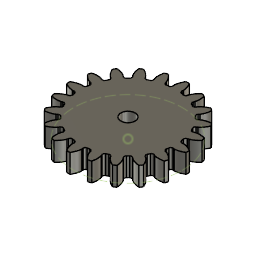
gear (Autodesk Fusion 360 design; units mm, degrees)
description: Spur Gear; Module: 2.000000; Num Teeth: 20; Pressure Angle: 20.000000; Backlash: 0.20 mm
Autodesk Fusion 360 part; units mm, degrees
(part 1 of 3)
sketch "Sketch1" plane through (0, 0, 0) normal (0, 0, 1) x (1, 0, 0) in component "Spur Gear (20 teeth)"
  circle A0 centre (0, 0) radius 17.5492
extrude "Extrude1" add sketch "Sketch1" along normal blind 7 in component "Spur Gear (20 teeth)"
sketch "Sketch2" plane through (0, 0, 0) normal (0, 0, 1) x (1, 0, 0) in component "Spur Gear (20 teeth)"
  spline S0 degree 5 poles (18.7162, -1.7068) (18.7256, -1.7077) (18.7444, -1.7091) (18.7726, -1.7106) (18.8102, -1.7111) (18.8573, -1.7097) (18.9045, -1.707) (18.9518, -1.7034) (18.999, -1.6994) (19.0463, -1.695) (19.0936, -1.6902) (19.1409, -1.6851) (19.1883, -1.6793) (19.2356, -1.6729) (19.2829, -1.6658) (19.3303, -1.658) (19.3776, -1.6497) (19.425, -1.641) (19.4723, -1.6318) (19.5197, -1.6223) (19.567, -1.6124) (19.6143, -1.6021) (19.6616, -1.5914) (19.7089, -1.5802) (19.7562, -1.5687) (19.8035, -1.5567) (19.8507, -1.5444) (19.898, -1.5316) (19.9452, -1.5186) (19.9924, -1.5051) (20.0396, -1.4914) (20.0867, -1.4773) (20.1339, -1.4628) (20.181, -1.448) (20.2281, -1.4329) (20.2752, -1.4174) (20.3222, -1.4016) (20.3692, -1.3854) (20.4162, -1.369) (20.4631, -1.3523) (20.5101, -1.3352) (20.557, -1.3178) (20.6038, -1.3001) (20.6506, -1.2822) (20.6974, -1.2639) (20.7442, -1.2453) (20.7909, -1.2264) (20.8376, -1.2073) (20.8843, -1.1878) (20.9309, -1.1681) (20.9774, -1.1481) (21.024, -1.1278) (21.0705, -1.1072) (21.1169, -1.0863) (21.1633, -1.0652) (21.2097, -1.0438) (21.256, -1.0221) (21.3023, -1.0002) (21.3485, -0.978) (21.3947, -0.9555) (21.4409, -0.9328) (21.487, -0.9098) (21.533, -0.8865) (21.579, -0.863) (21.625, -0.8392) (21.6709, -0.8151) (21.7167, -0.7909) (21.7625, -0.7663) (21.8083, -0.7415) (21.8539, -0.7165) (21.8996, -0.6912) (21.9361, -0.6707) (21.9634, -0.6553) (21.9816, -0.645) (21.9907, -0.6398) knots 0 0 0 0 0 0 0.01428571 0.02857143 0.04285714 0.05714286 0.07142857 0.08571429 0.1 0.11428571 0.12857143 0.14285714 0.15714286 0.17142857 0.18571429 0.2 0.21428571 0.22857143 0.24285714 0.25714286 0.27142857 0.28571429 0.3 0.31428571 0.32857143 0.34285714 0.35714286 0.37142857 0.38571429 0.4 0.41428571 0.42857143 0.44285714 0.45714286 0.47142857 0.48571429 0.5 0.51428571 0.52857143 0.54285714 0.55714286 0.57142857 0.58571429 0.6 0.61428571 0.62857143 0.64285714 0.65714286 0.67142857 0.68571429 0.7 0.71428571 0.72857143 0.74285714 0.75714286 0.77142857 0.78571429 0.8 0.81428571 0.82857143 0.84285714 0.85714286 0.87142857 0.88571429 0.9 0.91428571 0.92857143 0.94285714 0.95714286 0.97142857 0.98571429 1 1 1 1 1 1
  spline S1 degree 5 poles (18.7162, 1.7068) (18.7256, 1.7077) (18.7444, 1.7091) (18.7726, 1.7106) (18.8102, 1.7111) (18.8573, 1.7097) (18.9045, 1.707) (18.9518, 1.7034) (18.999, 1.6994) (19.0463, 1.695) (19.0936, 1.6902) (19.1409, 1.6851) (19.1883, 1.6793) (19.2356, 1.6729) (19.2829, 1.6658) (19.3303, 1.658) (19.3776, 1.6497) (19.425, 1.641) (19.4723, 1.6318) (19.5197, 1.6223) (19.567, 1.6124) (19.6143, 1.6021) (19.6616, 1.5914) (19.7089, 1.5802) (19.7562, 1.5687) (19.8035, 1.5567) (19.8507, 1.5444) (19.898, 1.5316) (19.9452, 1.5186) (19.9924, 1.5051) (20.0396, 1.4914) (20.0867, 1.4773) (20.1339, 1.4628) (20.181, 1.448) (20.2281, 1.4329) (20.2752, 1.4174) (20.3222, 1.4016) (20.3692, 1.3854) (20.4162, 1.369) (20.4631, 1.3523) (20.5101, 1.3352) (20.557, 1.3178) (20.6038, 1.3001) (20.6506, 1.2822) (20.6974, 1.2639) (20.7442, 1.2453) (20.7909, 1.2264) (20.8376, 1.2073) (20.8843, 1.1878) (20.9309, 1.1681) (20.9774, 1.1481) (21.024, 1.1278) (21.0705, 1.1072) (21.1169, 1.0863) (21.1633, 1.0652) (21.2097, 1.0438) (21.256, 1.0221) (21.3023, 1.0002) (21.3485, 0.978) (21.3947, 0.9555) (21.4409, 0.9328) (21.487, 0.9098) (21.533, 0.8865) (21.579, 0.863) (21.625, 0.8392) (21.6709, 0.8151) (21.7167, 0.7909) (21.7625, 0.7663) (21.8083, 0.7415) (21.8539, 0.7165) (21.8996, 0.6912) (21.9361, 0.6707) (21.9634, 0.6553) (21.9816, 0.645) (21.9907, 0.6398) knots 0 0 0 0 0 0 0.01428571 0.02857143 0.04285714 0.05714286 0.07142857 0.08571429 0.1 0.11428571 0.12857143 0.14285714 0.15714286 0.17142857 0.18571429 0.2 0.21428571 0.22857143 0.24285714 0.25714286 0.27142857 0.28571429 0.3 0.31428571 0.32857143 0.34285714 0.35714286 0.37142857 0.38571429 0.4 0.41428571 0.42857143 0.44285714 0.45714286 0.47142857 0.48571429 0.5 0.51428571 0.52857143 0.54285714 0.55714286 0.57142857 0.58571429 0.6 0.61428571 0.62857143 0.64285714 0.65714286 0.67142857 0.68571429 0.7 0.71428571 0.72857143 0.74285714 0.75714286 0.77142857 0.78571429 0.8 0.81428571 0.82857143 0.84285714 0.85714286 0.87142857 0.88571429 0.9 0.91428571 0.92857143 0.94285714 0.95714286 0.97142857 0.98571429 1 1 1 1 1 1
  arc A0 (21.9907, -0.6398) -> (21.9907, 0.6398) centre (0, 0) ccw
  line L0 (17.4667, -1.5938) -> (18.7162, -1.7068)
  line L1 (17.4667, 1.5938) -> (18.7162, 1.7068)
  line L2 (17.4667, -1.5938) -> (17.4667, 1.5938)
  point P0 (18.9464, -1.7037)
  point P1 (19.1784, -1.6804)
  point P2 (19.4114, -1.6434)
  point P3 (19.6452, -1.595)
  point P4 (19.8796, -1.5365)
  point P5 (20.1144, -1.4687)
  point P6 (20.3494, -1.3922)
  point P7 (20.5845, -1.3074)
  point P8 (20.8195, -1.2147)
  point P9 (21.0545, -1.1142)
  point P10 (21.2892, -1.0064)
  point P11 (21.5235, -0.8912)
  point P12 (21.7574, -0.769)
  point P13 (18.9464, 1.7037)
  point P14 (19.1784, 1.6804)
  point P15 (19.4114, 1.6434)
  point P16 (19.6452, 1.595)
  point P17 (19.8796, 1.5365)
  point P18 (20.1144, 1.4687)
  point P19 (20.3494, 1.3922)
  point P20 (20.5845, 1.3074)
  point P21 (20.8195, 1.2147)
  point P22 (21.0545, 1.1142)
  point P23 (21.2892, 1.0064)
  point P24 (21.5235, 0.8912)
  point P25 (21.7574, 0.769)
extrude "Extrude2" add sketch "Sketch2" along normal blind 7 in component "Spur Gear (20 teeth)"
fillet "Fillet1" radius 0.75 2 edges at (17.4766, -1.5947, 3.5) (17.4766, 1.5947, 3.5) in component "Spur Gear (20 teeth)"
pattern_circular "C-Pattern1" count 20 over 360 about axis through (0, 0, 0) along (0, 0, 1) of "Extrude2", "Fillet1" in component "Spur Gear (20 teeth)"
sketch "Sketch3" plane through (0, 0, 0) normal (0, 0, 1) x (1, 0, 0) in component "Spur Gear (20 teeth)"
  circle A0 centre (0, 0) radius 20 construction
sketch "Sketch1 (2)" plane through (0, 0, 7) normal (0, 0, 1) x (-1, 0, 0)
  arc A0 (-17.2587, 3.1798) -> (-17.3966, 2.3091) centre (0, 0) ccw
  arc A1 (-18.2077, 1.6608) -> (-17.3966, 2.3091) centre (-18.1401, 2.4078) ccw
  line L0 (-18.2077, 1.6608) -> (-18.7162, 1.7068)
  spline S0 degree 5 poles (-18.7162, 1.7068) (-18.7256, 1.7077) (-18.7444, 1.7091) (-18.7726, 1.7106) (-18.8102, 1.7111) (-18.8573, 1.7097) (-18.9045, 1.707) (-18.9518, 1.7034) (-18.999, 1.6994) (-19.0463, 1.695) (-19.0936, 1.6902) (-19.1409, 1.6851) (-19.1883, 1.6793) (-19.2356, 1.6729) (-19.2829, 1.6658) (-19.3303, 1.658) (-19.3776, 1.6497) (-19.425, 1.641) (-19.4723, 1.6318) (-19.5197, 1.6223) (-19.567, 1.6124) (-19.6143, 1.6021) (-19.6616, 1.5914) (-19.7089, 1.5802) (-19.7562, 1.5687) (-19.8035, 1.5567) (-19.8507, 1.5444) (-19.898, 1.5316) (-19.9452, 1.5186) (-19.9924, 1.5051) (-20.0396, 1.4914) (-20.0867, 1.4773) (-20.1339, 1.4628) (-20.181, 1.448) (-20.2281, 1.4329) (-20.2752, 1.4174) (-20.3222, 1.4016) (-20.3692, 1.3854) (-20.4162, 1.369) (-20.4631, 1.3523) (-20.5101, 1.3352) (-20.557, 1.3178) (-20.6038, 1.3001) (-20.6506, 1.2822) (-20.6974, 1.2639) (-20.7442, 1.2453) (-20.7909, 1.2264) (-20.8376, 1.2073) (-20.8843, 1.1878) (-20.9309, 1.1681) (-20.9774, 1.1481) (-21.024, 1.1278) (-21.0705, 1.1072) (-21.1169, 1.0863) (-21.1633, 1.0652) (-21.2097, 1.0438) (-21.256, 1.0221) (-21.3023, 1.0002) (-21.3485, 0.978) (-21.3947, 0.9555) (-21.4409, 0.9328) (-21.487, 0.9098) (-21.533, 0.8865) (-21.579, 0.863) (-21.625, 0.8392) (-21.6709, 0.8151) (-21.7167, 0.7909) (-21.7625, 0.7663) (-21.8083, 0.7415) (-21.8539, 0.7165) (-21.8996, 0.6912) (-21.9361, 0.6707) (-21.9634, 0.6553) (-21.9816, 0.645) (-21.9907, 0.6398) knots 0 0 0 0 0 0 0.01428571 0.02857143 0.04285714 0.05714286 0.07142857 0.08571429 0.1 0.11428571 0.12857143 0.14285714 0.15714286 0.17142857 0.18571429 0.2 0.21428571 0.22857143 0.24285714 0.25714286 0.27142857 0.28571429 0.3 0.31428571 0.32857143 0.34285714 0.35714286 0.37142857 0.38571429 0.4 0.41428571 0.42857143 0.44285714 0.45714286 0.47142857 0.48571429 0.5 0.51428571 0.52857143 0.54285714 0.55714286 0.57142857 0.58571429 0.6 0.61428571 0.62857143 0.64285714 0.65714286 0.67142857 0.68571429 0.7 0.71428571 0.72857143 0.74285714 0.75714286 0.77142857 0.78571429 0.8 0.81428571 0.82857143 0.84285714 0.85714286 0.87142857 0.88571429 0.9 0.91428571 0.92857143 0.94285714 0.95714286 0.97142857 0.98571429 1 1 1 1 1 1
  arc A2 (-21.9907, 0.6398) -> (-21.9907, -0.6398) centre (0, 0) ccw
  spline S1 degree 5 poles (-21.9907, -0.6398) (-21.9816, -0.645) (-21.9634, -0.6553) (-21.9361, -0.6707) (-21.8996, -0.6912) (-21.8539, -0.7165) (-21.8083, -0.7415) (-21.7625, -0.7663) (-21.7167, -0.7909) (-21.6709, -0.8151) (-21.625, -0.8392) (-21.579, -0.863) (-21.533, -0.8865) (-21.487, -0.9098) (-21.4409, -0.9328) (-21.3947, -0.9555) (-21.3485, -0.978) (-21.3023, -1.0002) (-21.256, -1.0221) (-21.2097, -1.0438) (-21.1633, -1.0652) (-21.1169, -1.0863) (-21.0705, -1.1072) (-21.024, -1.1278) (-20.9774, -1.1481) (-20.9309, -1.1681) (-20.8843, -1.1878) (-20.8376, -1.2073) (-20.7909, -1.2264) (-20.7442, -1.2453) (-20.6974, -1.2639) (-20.6506, -1.2822) (-20.6038, -1.3001) (-20.557, -1.3178) (-20.5101, -1.3352) (-20.4631, -1.3523) (-20.4162, -1.369) (-20.3692, -1.3854) (-20.3222, -1.4016) (-20.2752, -1.4174) (-20.2281, -1.4329) (-20.181, -1.448) (-20.1339, -1.4628) (-20.0867, -1.4773) (-20.0396, -1.4914) (-19.9924, -1.5051) (-19.9452, -1.5186) (-19.898, -1.5316) (-19.8507, -1.5444) (-19.8035, -1.5567) (-19.7562, -1.5687) (-19.7089, -1.5802) (-19.6616, -1.5914) (-19.6143, -1.6021) (-19.567, -1.6124) (-19.5197, -1.6223) (-19.4723, -1.6318) (-19.425, -1.641) (-19.3776, -1.6497) (-19.3303, -1.658) (-19.2829, -1.6658) (-19.2356, -1.6729) (-19.1883, -1.6793) (-19.1409, -1.6851) (-19.0936, -1.6902) (-19.0463, -1.695) (-18.999, -1.6994) (-18.9518, -1.7034) (-18.9045, -1.707) (-18.8573, -1.7097) (-18.8102, -1.7111) (-18.7726, -1.7106) (-18.7444, -1.7091) (-18.7256, -1.7077) (-18.7162, -1.7068) knots -1 -1 -1 -1 -1 -1 -0.98571429 -0.97142857 -0.95714286 -0.94285714 -0.92857143 -0.91428571 -0.9 -0.88571429 -0.87142857 -0.85714286 -0.84285714 -0.82857143 -0.81428571 -0.8 -0.78571429 -0.77142857 -0.75714286 -0.74285714 -0.72857143 -0.71428571 -0.7 -0.68571429 -0.67142857 -0.65714286 -0.64285714 -0.62857143 -0.61428571 -0.6 -0.58571429 -0.57142857 -0.55714286 -0.54285714 -0.52857143 -0.51428571 -0.5 -0.48571429 -0.47142857 -0.45714286 -0.44285714 -0.42857143 -0.41428571 -0.4 -0.38571429 -0.37142857 -0.35714286 -0.34285714 -0.32857143 -0.31428571 -0.3 -0.28571429 -0.27142857 -0.25714286 -0.24285714 -0.22857143 -0.21428571 -0.2 -0.18571429 -0.17142857 -0.15714286 -0.14285714 -0.12857143 -0.11428571 -0.1 -0.08571429 -0.07142857 -0.05714286 -0.04285714 -0.02857143 -0.01428571 0 0 0 0 0 0
  line L1 (-18.7162, -1.7068) -> (-18.2077, -1.6608)
  arc A3 (-17.3966, -2.3091) -> (-18.2077, -1.6608) centre (-18.1401, -2.4078) ccw
  arc A4 (-17.3966, -2.3091) -> (-17.2587, -3.1798) centre (0, 0) ccw
  arc A5 (-17.8298, -4.0469) -> (-17.2587, -3.1798) centre (-17.9963, -3.3157) ccw
  line L2 (-17.8298, -4.0469) -> (-18.3276, -4.1603)
  spline S2 degree 5 poles (-18.3276, -4.1603) (-18.3368, -4.1624) (-18.3551, -4.1668) (-18.3824, -4.1742) (-18.4183, -4.1854) (-18.4627, -4.2012) (-18.5068, -4.2183) (-18.5506, -4.2364) (-18.5943, -4.2548) (-18.6379, -4.2736) (-18.6814, -4.2927) (-18.7248, -4.3123) (-18.7681, -4.3324) (-18.8111, -4.3531) (-18.8539, -4.3745) (-18.8966, -4.3965) (-18.939, -4.419) (-18.9813, -4.442) (-19.0235, -4.4653) (-19.0656, -4.489) (-19.1076, -4.5131) (-19.1494, -4.5375) (-19.1911, -4.5623) (-19.2326, -4.5875) (-19.274, -4.6131) (-19.3153, -4.6391) (-19.3564, -4.6654) (-19.3974, -4.6921) (-19.4383, -4.7192) (-19.479, -4.7465) (-19.5196, -4.7742) (-19.5601, -4.8022) (-19.6005, -4.8305) (-19.6407, -4.8592) (-19.6808, -4.8881) (-19.7208, -4.9174) (-19.7607, -4.9469) (-19.8004, -4.9768) (-19.84, -5.0069) (-19.8795, -5.0374) (-19.9188, -5.0681) (-19.9581, -5.0991) (-19.9972, -5.1304) (-20.0361, -5.162) (-20.075, -5.1938) (-20.1137, -5.2259) (-20.1523, -5.2583) (-20.1908, -5.291) (-20.2292, -5.3239) (-20.2674, -5.3571) (-20.3055, -5.3905) (-20.3435, -5.4242) (-20.3813, -5.4581) (-20.4191, -5.4923) (-20.4567, -5.5267) (-20.4942, -5.5614) (-20.5315, -5.5964) (-20.5688, -5.6315) (-20.6059, -5.6669) (-20.6429, -5.7026) (-20.6797, -5.7385) (-20.7164, -5.7746) (-20.753, -5.811) (-20.7895, -5.8476) (-20.8259, -5.8844) (-20.8621, -5.9214) (-20.8982, -5.9587) (-20.9342, -5.9962) (-20.97, -6.0339) (-21.0057, -6.0718) (-21.0413, -6.11) (-21.0697, -6.1407) (-21.0909, -6.1638) (-21.105, -6.1793) (-21.1121, -6.187) knots 0 0 0 0 0 0 0.01428571 0.02857143 0.04285714 0.05714286 0.07142857 0.08571429 0.1 0.11428571 0.12857143 0.14285714 0.15714286 0.17142857 0.18571429 0.2 0.21428571 0.22857143 0.24285714 0.25714286 0.27142857 0.28571429 0.3 0.31428571 0.32857143 0.34285714 0.35714286 0.37142857 0.38571429 0.4 0.41428571 0.42857143 0.44285714 0.45714286 0.47142857 0.48571429 0.5 0.51428571 0.52857143 0.54285714 0.55714286 0.57142857 0.58571429 0.6 0.61428571 0.62857143 0.64285714 0.65714286 0.67142857 0.68571429 0.7 0.71428571 0.72857143 0.74285714 0.75714286 0.77142857 0.78571429 0.8 0.81428571 0.82857143 0.84285714 0.85714286 0.87142857 0.88571429 0.9 0.91428571 0.92857143 0.94285714 0.95714286 0.97142857 0.98571429 1 1 1 1 1 1
  arc A6 (-21.1121, -6.187) -> (-20.7167, -7.404) centre (0, 0) ccw
  spline S3 degree 5 poles (-20.7167, -7.404) (-20.7064, -7.4061) (-20.6859, -7.4103) (-20.6552, -7.4165) (-20.6142, -7.4247) (-20.5629, -7.4346) (-20.5117, -7.4443) (-20.4606, -7.4538) (-20.4094, -7.463) (-20.3583, -7.4719) (-20.3072, -7.4806) (-20.2562, -7.489) (-20.2052, -7.4972) (-20.1542, -7.5051) (-20.1032, -7.5127) (-20.0523, -7.5201) (-20.0014, -7.5272) (-19.9506, -7.534) (-19.8998, -7.5406) (-19.8491, -7.5469) (-19.7983, -7.5529) (-19.7477, -7.5587) (-19.6971, -7.5641) (-19.6465, -7.5693) (-19.5959, -7.5743) (-19.5455, -7.5789) (-19.495, -7.5833) (-19.4447, -7.5874) (-19.3943, -7.5912) (-19.3441, -7.5947) (-19.2939, -7.5979) (-19.2437, -7.6008) (-19.1936, -7.6034) (-19.1436, -7.6058) (-19.0936, -7.6078) (-19.0437, -7.6095) (-18.9939, -7.611) (-18.9441, -7.6121) (-18.8944, -7.6129) (-18.8448, -7.6134) (-18.7953, -7.6135) (-18.7458, -7.6134) (-18.6964, -7.6129) (-18.6471, -7.6121) (-18.5979, -7.6109) (-18.5488, -7.6095) (-18.4998, -7.6076) (-18.4508, -7.6055) (-18.4019, -7.603) (-18.3532, -7.6001) (-18.3045, -7.5969) (-18.256, -7.5933) (-18.2076, -7.5893) (-18.1592, -7.5848) (-18.1111, -7.58) (-18.063, -7.5748) (-18.015, -7.5692) (-17.9672, -7.5633) (-17.9194, -7.557) (-17.8718, -7.5503) (-17.8244, -7.543) (-17.7772, -7.5351) (-17.7302, -7.5266) (-17.6834, -7.5175) (-17.6368, -7.5078) (-17.5904, -7.4976) (-17.544, -7.4872) (-17.4978, -7.4765) (-17.4518, -7.4653) (-17.4061, -7.4533) (-17.3608, -7.44) (-17.3252, -7.4279) (-17.2988, -7.4178) (-17.2814, -7.4106) (-17.2727, -7.4069) knots -1 -1 -1 -1 -1 -1 -0.98571429 -0.97142857 -0.95714286 -0.94285714 -0.92857143 -0.91428571 -0.9 -0.88571429 -0.87142857 -0.85714286 -0.84285714 -0.82857143 -0.81428571 -0.8 -0.78571429 -0.77142857 -0.75714286 -0.74285714 -0.72857143 -0.71428571 -0.7 -0.68571429 -0.67142857 -0.65714286 -0.64285714 -0.62857143 -0.61428571 -0.6 -0.58571429 -0.57142857 -0.55714286 -0.54285714 -0.52857143 -0.51428571 -0.5 -0.48571429 -0.47142857 -0.45714286 -0.44285714 -0.42857143 -0.41428571 -0.4 -0.38571429 -0.37142857 -0.35714286 -0.34285714 -0.32857143 -0.31428571 -0.3 -0.28571429 -0.27142857 -0.25714286 -0.24285714 -0.22857143 -0.21428571 -0.2 -0.18571429 -0.17142857 -0.15714286 -0.14285714 -0.12857143 -0.11428571 -0.1 -0.08571429 -0.07142857 -0.05714286 -0.04285714 -0.02857143 -0.01428571 0 0 0 0 0 0
  line L3 (-17.2727, -7.4069) -> (-16.8033, -7.206)
  arc A7 (-15.8316, -7.5719) -> (-16.8033, -7.206) centre (-16.5082, -7.8955) ccw
  arc A8 (-15.8316, -7.5719) -> (-15.4314, -8.3574) centre (0, 0) ccw
  arc A9 (-15.7065, -9.3586) -> (-15.4314, -8.3574) centre (-16.0909, -8.7145) ccw
  line L4 (-15.7065, -9.3586) -> (-16.145, -9.6202)
  spline S4 degree 5 poles (-16.145, -9.6202) (-16.1531, -9.6251) (-16.1691, -9.6349) (-16.1928, -9.6504) (-16.2235, -9.6721) (-16.2609, -9.7009) (-16.2974, -9.7308) (-16.3336, -9.7615) (-16.3694, -9.7925) (-16.4051, -9.8239) (-16.4406, -9.8555) (-16.4758, -9.8875) (-16.5107, -9.92) (-16.5452, -9.953) (-16.5793, -9.9866) (-16.6131, -10.0207) (-16.6465, -10.0552) (-16.6797, -10.0902) (-16.7126, -10.1254) (-16.7453, -10.1609) (-16.7778, -10.1967) (-16.81, -10.2329) (-16.842, -10.2694) (-16.8737, -10.3062) (-16.9052, -10.3433) (-16.9364, -10.3808) (-16.9673, -10.4186) (-16.9981, -10.4566) (-17.0286, -10.495) (-17.0589, -10.5336) (-17.089, -10.5724) (-17.1188, -10.6116) (-17.1485, -10.651) (-17.1779, -10.6906) (-17.2071, -10.7306) (-17.2361, -10.7708) (-17.2648, -10.8112) (-17.2934, -10.8519) (-17.3217, -10.8928) (-17.3499, -10.9339) (-17.3778, -10.9753) (-17.4055, -11.0169) (-17.433, -11.0588) (-17.4604, -11.1008) (-17.4875, -11.1431) (-17.5144, -11.1857) (-17.5411, -11.2284) (-17.5676, -11.2713) (-17.5939, -11.3145) (-17.62, -11.3578) (-17.6459, -11.4014) (-17.6716, -11.4452) (-17.6972, -11.4892) (-17.7225, -11.5333) (-17.7476, -11.5777) (-17.7725, -11.6223) (-17.7973, -11.667) (-17.8218, -11.712) (-17.8462, -11.7572) (-17.8703, -11.8025) (-17.8943, -11.848) (-17.9181, -11.8937) (-17.9416, -11.9396) (-17.965, -11.9857) (-17.9882, -12.0319) (-18.0112, -12.0783) (-18.034, -12.1249) (-18.0567, -12.1717) (-18.0791, -12.2187) (-18.1013, -12.2658) (-18.1234, -12.3131) (-18.1409, -12.351) (-18.1539, -12.3796) (-18.1626, -12.3987) (-18.1669, -12.4082) knots 0 0 0 0 0 0 0.01428571 0.02857143 0.04285714 0.05714286 0.07142857 0.08571429 0.1 0.11428571 0.12857143 0.14285714 0.15714286 0.17142857 0.18571429 0.2 0.21428571 0.22857143 0.24285714 0.25714286 0.27142857 0.28571429 0.3 0.31428571 0.32857143 0.34285714 0.35714286 0.37142857 0.38571429 0.4 0.41428571 0.42857143 0.44285714 0.45714286 0.47142857 0.48571429 0.5 0.51428571 0.52857143 0.54285714 0.55714286 0.57142857 0.58571429 0.6 0.61428571 0.62857143 0.64285714 0.65714286 0.67142857 0.68571429 0.7 0.71428571 0.72857143 0.74285714 0.75714286 0.77142857 0.78571429 0.8 0.81428571 0.82857143 0.84285714 0.85714286 0.87142857 0.88571429 0.9 0.91428571 0.92857143 0.94285714 0.95714286 0.97142857 0.98571429 1 1 1 1 1 1
  arc A10 (-18.1669, -12.4082) -> (-17.4148, -13.4434) centre (0, 0) ccw
  spline S5 degree 5 poles (-17.4148, -13.4434) (-17.4044, -13.4422) (-17.3836, -13.4399) (-17.3524, -13.4363) (-17.3109, -13.4314) (-17.2591, -13.4251) (-17.2074, -13.4185) (-17.1558, -13.4116) (-17.1043, -13.4046) (-17.053, -13.3973) (-17.0017, -13.3897) (-16.9505, -13.382) (-16.8995, -13.374) (-16.8486, -13.3657) (-16.7978, -13.3572) (-16.7471, -13.3485) (-16.6965, -13.3395) (-16.646, -13.3303) (-16.5957, -13.3209) (-16.5455, -13.3112) (-16.4954, -13.3013) (-16.4454, -13.2911) (-16.3956, -13.2807) (-16.3459, -13.27) (-16.2963, -13.259) (-16.2468, -13.2479) (-16.1975, -13.2364) (-16.1484, -13.2247) (-16.0993, -13.2128) (-16.0504, -13.2006) (-16.0017, -13.1882) (-15.9531, -13.1754) (-15.9046, -13.1625) (-15.8563, -13.1492) (-15.8082, -13.1357) (-15.7602, -13.1219) (-15.7124, -13.1079) (-15.6647, -13.0936) (-15.6172, -13.079) (-15.5698, -13.0641) (-15.5227, -13.049) (-15.4757, -13.0335) (-15.4288, -13.0178) (-15.3822, -13.0018) (-15.3358, -12.9855) (-15.2895, -12.9689) (-15.2434, -12.952) (-15.1975, -12.9349) (-15.1518, -12.9174) (-15.1063, -12.8996) (-15.0611, -12.8815) (-15.016, -12.8631) (-14.9712, -12.8443) (-14.9266, -12.8251) (-14.8823, -12.8056) (-14.8382, -12.7858) (-14.7943, -12.7657) (-14.7506, -12.7453) (-14.7072, -12.7245) (-14.664, -12.7034) (-14.6211, -12.6819) (-14.5786, -12.6598) (-14.5366, -12.6372) (-14.4949, -12.614) (-14.4536, -12.5904) (-14.4125, -12.5664) (-14.3717, -12.5422) (-14.331, -12.5177) (-14.2907, -12.4928) (-14.2509, -12.4673) (-14.212, -12.4406) (-14.1819, -12.4181) (-14.1599, -12.4004) (-14.1456, -12.3882) (-14.1385, -12.382) knots -1 -1 -1 -1 -1 -1 -0.98571429 -0.97142857 -0.95714286 -0.94285714 -0.92857143 -0.91428571 -0.9 -0.88571429 -0.87142857 -0.85714286 -0.84285714 -0.82857143 -0.81428571 -0.8 -0.78571429 -0.77142857 -0.75714286 -0.74285714 -0.72857143 -0.71428571 -0.7 -0.68571429 -0.67142857 -0.65714286 -0.64285714 -0.62857143 -0.61428571 -0.6 -0.58571429 -0.57142857 -0.55714286 -0.54285714 -0.52857143 -0.51428571 -0.5 -0.48571429 -0.47142857 -0.45714286 -0.44285714 -0.42857143 -0.41428571 -0.4 -0.38571429 -0.37142857 -0.35714286 -0.34285714 -0.32857143 -0.31428571 -0.3 -0.28571429 -0.27142857 -0.25714286 -0.24285714 -0.22857143 -0.21428571 -0.2 -0.18571429 -0.17142857 -0.15714286 -0.14285714 -0.12857143 -0.11428571 -0.1 -0.08571429 -0.07142857 -0.05714286 -0.04285714 -0.02857143 -0.01428571 0 0 0 0 0 0
  line L5 (-14.1385, -12.382) -> (-13.7541, -12.0458)
  arc A11 (-12.7169, -12.0936) -> (-13.7541, -12.0458) centre (-13.2604, -12.6104) ccw
  arc A12 (-12.7169, -12.0936) -> (-12.0936, -12.7169) centre (0, 0) ccw
  arc A13 (-12.0458, -13.7541) -> (-12.0936, -12.7169) centre (-12.6104, -13.2604) ccw
  line L6 (-12.0458, -13.7541) -> (-12.382, -14.1385)
  spline S6 degree 5 poles (-12.382, -14.1385) (-12.3882, -14.1456) (-12.4004, -14.1599) (-12.4181, -14.1819) (-12.4406, -14.212) (-12.4673, -14.2509) (-12.4928, -14.2907) (-12.5177, -14.331) (-12.5422, -14.3717) (-12.5664, -14.4125) (-12.5904, -14.4536) (-12.614, -14.4949) (-12.6372, -14.5366) (-12.6598, -14.5786) (-12.6819, -14.6211) (-12.7034, -14.664) (-12.7245, -14.7072) (-12.7453, -14.7506) (-12.7657, -14.7943) (-12.7858, -14.8382) (-12.8056, -14.8823) (-12.8251, -14.9266) (-12.8443, -14.9712) (-12.8631, -15.016) (-12.8815, -15.0611) (-12.8996, -15.1063) (-12.9174, -15.1518) (-12.9349, -15.1975) (-12.952, -15.2434) (-12.9689, -15.2895) (-12.9855, -15.3358) (-13.0018, -15.3822) (-13.0178, -15.4288) (-13.0335, -15.4757) (-13.049, -15.5227) (-13.0641, -15.5698) (-13.079, -15.6172) (-13.0936, -15.6647) (-13.1079, -15.7124) (-13.1219, -15.7602) (-13.1357, -15.8082) (-13.1492, -15.8563) (-13.1625, -15.9046) (-13.1754, -15.9531) (-13.1882, -16.0017) (-13.2006, -16.0504) (-13.2128, -16.0993) (-13.2247, -16.1484) (-13.2364, -16.1975) (-13.2479, -16.2468) (-13.259, -16.2963) (-13.27, -16.3459) (-13.2807, -16.3956) (-13.2911, -16.4454) (-13.3013, -16.4954) (-13.3112, -16.5455) (-13.3209, -16.5957) (-13.3303, -16.646) (-13.3395, -16.6965) (-13.3485, -16.7471) (-13.3572, -16.7978) (-13.3657, -16.8486) (-13.374, -16.8995) (-13.382, -16.9505) (-13.3897, -17.0017) (-13.3973, -17.053) (-13.4046, -17.1043) (-13.4116, -17.1558) (-13.4185, -17.2074) (-13.4251, -17.2591) (-13.4314, -17.3109) (-13.4363, -17.3524) (-13.4399, -17.3836) (-13.4422, -17.4044) (-13.4434, -17.4148) knots 0 0 0 0 0 0 0.01428571 0.02857143 0.04285714 0.05714286 0.07142857 0.08571429 0.1 0.11428571 0.12857143 0.14285714 0.15714286 0.17142857 0.18571429 0.2 0.21428571 0.22857143 0.24285714 0.25714286 0.27142857 0.28571429 0.3 0.31428571 0.32857143 0.34285714 0.35714286 0.37142857 0.38571429 0.4 0.41428571 0.42857143 0.44285714 0.45714286 0.47142857 0.48571429 0.5 0.51428571 0.52857143 0.54285714 0.55714286 0.57142857 0.58571429 0.6 0.61428571 0.62857143 0.64285714 0.65714286 0.67142857 0.68571429 0.7 0.71428571 0.72857143 0.74285714 0.75714286 0.77142857 0.78571429 0.8 0.81428571 0.82857143 0.84285714 0.85714286 0.87142857 0.88571429 0.9 0.91428571 0.92857143 0.94285714 0.95714286 0.97142857 0.98571429 1 1 1 1 1 1
  arc A14 (-13.4434, -17.4148) -> (-12.4082, -18.1669) centre (0, 0) ccw
  spline S7 degree 5 poles (-12.4082, -18.1669) (-12.3987, -18.1626) (-12.3796, -18.1539) (-12.351, -18.1409) (-12.3131, -18.1234) (-12.2658, -18.1013) (-12.2187, -18.0791) (-12.1717, -18.0567) (-12.1249, -18.034) (-12.0783, -18.0112) (-12.0319, -17.9882) (-11.9857, -17.965) (-11.9396, -17.9416) (-11.8937, -17.9181) (-11.848, -17.8943) (-11.8025, -17.8703) (-11.7572, -17.8462) (-11.712, -17.8218) (-11.667, -17.7973) (-11.6223, -17.7725) (-11.5777, -17.7476) (-11.5333, -17.7225) (-11.4892, -17.6972) (-11.4452, -17.6716) (-11.4014, -17.6459) (-11.3578, -17.62) (-11.3145, -17.5939) (-11.2713, -17.5676) (-11.2284, -17.5411) (-11.1857, -17.5144) (-11.1431, -17.4875) (-11.1008, -17.4604) (-11.0588, -17.433) (-11.0169, -17.4055) (-10.9753, -17.3778) (-10.9339, -17.3499) (-10.8928, -17.3217) (-10.8519, -17.2934) (-10.8112, -17.2648) (-10.7708, -17.2361) (-10.7306, -17.2071) (-10.6906, -17.1779) (-10.651, -17.1485) (-10.6116, -17.1188) (-10.5724, -17.089) (-10.5336, -17.0589) (-10.495, -17.0286) (-10.4566, -16.9981) (-10.4186, -16.9673) (-10.3808, -16.9364) (-10.3433, -16.9052) (-10.3062, -16.8737) (-10.2694, -16.842) (-10.2329, -16.81) (-10.1967, -16.7778) (-10.1609, -16.7453) (-10.1254, -16.7126) (-10.0902, -16.6797) (-10.0552, -16.6465) (-10.0207, -16.6131) (-9.9866, -16.5793) (-9.953, -16.5452) (-9.92, -16.5107) (-9.8875, -16.4758) (-9.8555, -16.4406) (-9.8239, -16.4051) (-9.7925, -16.3694) (-9.7615, -16.3336) (-9.7308, -16.2974) (-9.7009, -16.2609) (-9.6721, -16.2235) (-9.6504, -16.1928) (-9.6349, -16.1691) (-9.6251, -16.1531) (-9.6202, -16.145) knots -1 -1 -1 -1 -1 -1 -0.98571429 -0.97142857 -0.95714286 -0.94285714 -0.92857143 -0.91428571 -0.9 -0.88571429 -0.87142857 -0.85714286 -0.84285714 -0.82857143 -0.81428571 -0.8 -0.78571429 -0.77142857 -0.75714286 -0.74285714 -0.72857143 -0.71428571 -0.7 -0.68571429 -0.67142857 -0.65714286 -0.64285714 -0.62857143 -0.61428571 -0.6 -0.58571429 -0.57142857 -0.55714286 -0.54285714 -0.52857143 -0.51428571 -0.5 -0.48571429 -0.47142857 -0.45714286 -0.44285714 -0.42857143 -0.41428571 -0.4 -0.38571429 -0.37142857 -0.35714286 -0.34285714 -0.32857143 -0.31428571 -0.3 -0.28571429 -0.27142857 -0.25714286 -0.24285714 -0.22857143 -0.21428571 -0.2 -0.18571429 -0.17142857 -0.15714286 -0.14285714 -0.12857143 -0.11428571 -0.1 -0.08571429 -0.07142857 -0.05714286 -0.04285714 -0.02857143 -0.01428571 0 0 0 0 0 0
  line L7 (-9.6202, -16.145) -> (-9.3586, -15.7065)
  arc A15 (-8.3574, -15.4314) -> (-9.3586, -15.7065) centre (-8.7145, -16.0909) ccw
  arc A16 (-8.3574, -15.4314) -> (-7.5719, -15.8316) centre (0, 0) ccw
  arc A17 (-7.206, -16.8033) -> (-7.5719, -15.8316) centre (-7.8955, -16.5082) ccw
  line L8 (-7.206, -16.8033) -> (-7.4069, -17.2727)
  spline S8 degree 5 poles (-7.4069, -17.2727) (-7.4106, -17.2814) (-7.4178, -17.2988) (-7.4279, -17.3252) (-7.44, -17.3608) (-7.4533, -17.4061) (-7.4653, -17.4518) (-7.4765, -17.4978) (-7.4872, -17.544) (-7.4976, -17.5904) (-7.5078, -17.6368) (-7.5175, -17.6834) (-7.5266, -17.7302) (-7.5351, -17.7772) (-7.543, -17.8244) (-7.5503, -17.8718) (-7.557, -17.9194) (-7.5633, -17.9672) (-7.5692, -18.015) (-7.5748, -18.063) (-7.58, -18.1111) (-7.5848, -18.1592) (-7.5893, -18.2076) (-7.5933, -18.256) (-7.5969, -18.3045) (-7.6001, -18.3532) (-7.603, -18.4019) (-7.6055, -18.4508) (-7.6076, -18.4998) (-7.6095, -18.5488) (-7.6109, -18.5979) (-7.6121, -18.6471) (-7.6129, -18.6964) (-7.6134, -18.7458) (-7.6135, -18.7953) (-7.6134, -18.8448) (-7.6129, -18.8944) (-7.6121, -18.9441) (-7.611, -18.9939) (-7.6095, -19.0437) (-7.6078, -19.0936) (-7.6058, -19.1436) (-7.6034, -19.1936) (-7.6008, -19.2437) (-7.5979, -19.2939) (-7.5947, -19.3441) (-7.5912, -19.3943) (-7.5874, -19.4447) (-7.5833, -19.495) (-7.5789, -19.5455) (-7.5743, -19.5959) (-7.5693, -19.6465) (-7.5641, -19.6971) (-7.5587, -19.7477) (-7.5529, -19.7983) (-7.5469, -19.8491) (-7.5406, -19.8998) (-7.534, -19.9506) (-7.5272, -20.0014) (-7.5201, -20.0523) (-7.5127, -20.1032) (-7.5051, -20.1542) (-7.4972, -20.2052) (-7.489, -20.2562) (-7.4806, -20.3072) (-7.4719, -20.3583) (-7.463, -20.4094) (-7.4538, -20.4606) (-7.4443, -20.5117) (-7.4346, -20.5629) (-7.4247, -20.6142) (-7.4165, -20.6552) (-7.4103, -20.6859) (-7.4061, -20.7064) (-7.404, -20.7167) knots 0 0 0 0 0 0 0.01428571 0.02857143 0.04285714 0.05714286 0.07142857 0.08571429 0.1 0.11428571 0.12857143 0.14285714 0.15714286 0.17142857 0.18571429 0.2 0.21428571 0.22857143 0.24285714 0.25714286 0.27142857 0.28571429 0.3 0.31428571 0.32857143 0.34285714 0.35714286 0.37142857 0.38571429 0.4 0.41428571 0.42857143 0.44285714 0.45714286 0.47142857 0.48571429 0.5 0.51428571 0.52857143 0.54285714 0.55714286 0.57142857 0.58571429 0.6 0.61428571 0.62857143 0.64285714 0.65714286 0.67142857 0.68571429 0.7 0.71428571 0.72857143 0.74285714 0.75714286 0.77142857 0.78571429 0.8 0.81428571 0.82857143 0.84285714 0.85714286 0.87142857 0.88571429 0.9 0.91428571 0.92857143 0.94285714 0.95714286 0.97142857 0.98571429 1 1 1 1 1 1
  arc A18 (-7.404, -20.7167) -> (-6.187, -21.1121) centre (0, 0) ccw
  spline S9 degree 5 poles (-6.187, -21.1121) (-6.1793, -21.105) (-6.1638, -21.0909) (-6.1407, -21.0697) (-6.11, -21.0413) (-6.0718, -21.0057) (-6.0339, -20.97) (-5.9962, -20.9342) (-5.9587, -20.8982) (-5.9214, -20.8621) (-5.8844, -20.8259) (-5.8476, -20.7895) (-5.811, -20.753) (-5.7746, -20.7164) (-5.7385, -20.6797) (-5.7026, -20.6429) (-5.6669, -20.6059) (-5.6315, -20.5688) (-5.5964, -20.5315) (-5.5614, -20.4942) (-5.5267, -20.4567) (-5.4923, -20.4191) (-5.4581, -20.3813) (-5.4242, -20.3435) (-5.3905, -20.3055) (-5.3571, -20.2674) (-5.3239, -20.2292) (-5.291, -20.1908) (-5.2583, -20.1523) (-5.2259, -20.1137) (-5.1938, -20.075) (-5.162, -20.0361) (-5.1304, -19.9972) (-5.0991, -19.9581) (-5.0681, -19.9188) (-5.0374, -19.8795) (-5.0069, -19.84) (-4.9768, -19.8004) (-4.9469, -19.7607) (-4.9174, -19.7208) (-4.8881, -19.6808) (-4.8592, -19.6407) (-4.8305, -19.6005) (-4.8022, -19.5601) (-4.7742, -19.5196) (-4.7465, -19.479) (-4.7192, -19.4383) (-4.6921, -19.3974) (-4.6654, -19.3564) (-4.6391, -19.3153) (-4.6131, -19.274) (-4.5875, -19.2326) (-4.5623, -19.1911) (-4.5375, -19.1494) (-4.5131, -19.1076) (-4.489, -19.0656) (-4.4653, -19.0235) (-4.442, -18.9813) (-4.419, -18.939) (-4.3965, -18.8966) (-4.3745, -18.8539) (-4.3531, -18.8111) (-4.3324, -18.7681) (-4.3123, -18.7248) (-4.2927, -18.6814) (-4.2736, -18.6379) (-4.2548, -18.5943) (-4.2364, -18.5506) (-4.2183, -18.5068) (-4.2012, -18.4627) (-4.1854, -18.4183) (-4.1742, -18.3824) (-4.1668, -18.3551) (-4.1624, -18.3368) (-4.1603, -18.3276) knots -1 -1 -1 -1 -1 -1 -0.98571429 -0.97142857 -0.95714286 -0.94285714 -0.92857143 -0.91428571 -0.9 -0.88571429 -0.87142857 -0.85714286 -0.84285714 -0.82857143 -0.81428571 -0.8 -0.78571429 -0.77142857 -0.75714286 -0.74285714 -0.72857143 -0.71428571 -0.7 -0.68571429 -0.67142857 -0.65714286 -0.64285714 -0.62857143 -0.61428571 -0.6 -0.58571429 -0.57142857 -0.55714286 -0.54285714 -0.52857143 -0.51428571 -0.5 -0.48571429 -0.47142857 -0.45714286 -0.44285714 -0.42857143 -0.41428571 -0.4 -0.38571429 -0.37142857 -0.35714286 -0.34285714 -0.32857143 -0.31428571 -0.3 -0.28571429 -0.27142857 -0.25714286 -0.24285714 -0.22857143 -0.21428571 -0.2 -0.18571429 -0.17142857 -0.15714286 -0.14285714 -0.12857143 -0.11428571 -0.1 -0.08571429 -0.07142857 -0.05714286 -0.04285714 -0.02857143 -0.01428571 0 0 0 0 0 0
  line L9 (-4.1603, -18.3276) -> (-4.0469, -17.8298)
  arc A19 (-3.1798, -17.2587) -> (-4.0469, -17.8298) centre (-3.3157, -17.9963) ccw
  arc A20 (-3.1798, -17.2587) -> (-2.3091, -17.3966) centre (0, 0) ccw
  arc A21 (-1.6608, -18.2077) -> (-2.3091, -17.3966) centre (-2.4078, -18.1401) ccw
  line L10 (-1.6608, -18.2077) -> (-1.7068, -18.7162)
  spline S10 degree 5 poles (-1.7068, -18.7162) (-1.7077, -18.7256) (-1.7091, -18.7444) (-1.7106, -18.7726) (-1.7111, -18.8102) (-1.7097, -18.8573) (-1.707, -18.9045) (-1.7034, -18.9518) (-1.6994, -18.999) (-1.695, -19.0463) (-1.6902, -19.0936) (-1.6851, -19.1409) (-1.6793, -19.1883) (-1.6729, -19.2356) (-1.6658, -19.2829) (-1.658, -19.3303) (-1.6497, -19.3776) (-1.641, -19.425) (-1.6318, -19.4723) (-1.6223, -19.5197) (-1.6124, -19.567) (-1.6021, -19.6143) (-1.5914, -19.6616) (-1.5802, -19.7089) (-1.5687, -19.7562) (-1.5567, -19.8035) (-1.5444, -19.8507) (-1.5316, -19.898) (-1.5186, -19.9452) (-1.5051, -19.9924) (-1.4914, -20.0396) (-1.4773, -20.0867) (-1.4628, -20.1339) (-1.448, -20.181) (-1.4329, -20.2281) (-1.4174, -20.2752) (-1.4016, -20.3222) (-1.3854, -20.3692) (-1.369, -20.4162) (-1.3523, -20.4631) (-1.3352, -20.5101) (-1.3178, -20.557) (-1.3001, -20.6038) (-1.2822, -20.6506) (-1.2639, -20.6974) (-1.2453, -20.7442) (-1.2264, -20.7909) (-1.2073, -20.8376) (-1.1878, -20.8843) (-1.1681, -20.9309) (-1.1481, -20.9774) (-1.1278, -21.024) (-1.1072, -21.0705) (-1.0863, -21.1169) (-1.0652, -21.1633) (-1.0438, -21.2097) (-1.0221, -21.256) (-1.0002, -21.3023) (-0.978, -21.3485) (-0.9555, -21.3947) (-0.9328, -21.4409) (-0.9098, -21.487) (-0.8865, -21.533) (-0.863, -21.579) (-0.8392, -21.625) (-0.8151, -21.6709) (-0.7909, -21.7167) (-0.7663, -21.7625) (-0.7415, -21.8083) (-0.7165, -21.8539) (-0.6912, -21.8996) (-0.6707, -21.9361) (-0.6553, -21.9634) (-0.645, -21.9816) (-0.6398, -21.9907) knots 0 0 0 0 0 0 0.01428571 0.02857143 0.04285714 0.05714286 0.07142857 0.08571429 0.1 0.11428571 0.12857143 0.14285714 0.15714286 0.17142857 0.18571429 0.2 0.21428571 0.22857143 0.24285714 0.25714286 0.27142857 0.28571429 0.3 0.31428571 0.32857143 0.34285714 0.35714286 0.37142857 0.38571429 0.4 0.41428571 0.42857143 0.44285714 0.45714286 0.47142857 0.48571429 0.5 0.51428571 0.52857143 0.54285714 0.55714286 0.57142857 0.58571429 0.6 0.61428571 0.62857143 0.64285714 0.65714286 0.67142857 0.68571429 0.7 0.71428571 0.72857143 0.74285714 0.75714286 0.77142857 0.78571429 0.8 0.81428571 0.82857143 0.84285714 0.85714286 0.87142857 0.88571429 0.9 0.91428571 0.92857143 0.94285714 0.95714286 0.97142857 0.98571429 1 1 1 1 1 1
  arc A22 (-0.6398, -21.9907) -> (0.6398, -21.9907) centre (0, 0) ccw
  spline S11 degree 5 poles (0.6398, -21.9907) (0.645, -21.9816) (0.6553, -21.9634) (0.6707, -21.9361) (0.6912, -21.8996) (0.7165, -21.8539) (0.7415, -21.8083) (0.7663, -21.7625) (0.7909, -21.7167) (0.8151, -21.6709) (0.8392, -21.625) (0.863, -21.579) (0.8865, -21.533) (0.9098, -21.487) (0.9328, -21.4409) (0.9555, -21.3947) (0.978, -21.3485) (1.0002, -21.3023) (1.0221, -21.256) (1.0438, -21.2097) (1.0652, -21.1633) (1.0863, -21.1169) (1.1072, -21.0705) (1.1278, -21.024) (1.1481, -20.9774) (1.1681, -20.9309) (1.1878, -20.8843) (1.2073, -20.8376) (1.2264, -20.7909) (1.2453, -20.7442) (1.2639, -20.6974) (1.2822, -20.6506) (1.3001, -20.6038) (1.3178, -20.557) (1.3352, -20.5101) (1.3523, -20.4631) (1.369, -20.4162) (1.3854, -20.3692) (1.4016, -20.3222) (1.4174, -20.2752) (1.4329, -20.2281) (1.448, -20.181) (1.4628, -20.1339) (1.4773, -20.0867) (1.4914, -20.0396) (1.5051, -19.9924) (1.5186, -19.9452) (1.5316, -19.898) (1.5444, -19.8507) (1.5567, -19.8035) (1.5687, -19.7562) (1.5802, -19.7089) (1.5914, -19.6616) (1.6021, -19.6143) (1.6124, -19.567) (1.6223, -19.5197) (1.6318, -19.4723) (1.641, -19.425) (1.6497, -19.3776) (1.658, -19.3303) (1.6658, -19.2829) (1.6729, -19.2356) (1.6793, -19.1883) (1.6851, -19.1409) (1.6902, -19.0936) (1.695, -19.0463) (1.6994, -18.999) (1.7034, -18.9518) (1.707, -18.9045) (1.7097, -18.8573) (1.7111, -18.8102) (1.7106, -18.7726) (1.7091, -18.7444) (1.7077, -18.7256) (1.7068, -18.7162) knots -1 -1 -1 -1 -1 -1 -0.98571429 -0.97142857 -0.95714286 -0.94285714 -0.92857143 -0.91428571 -0.9 -0.88571429 -0.87142857 -0.85714286 -0.84285714 -0.82857143 -0.81428571 -0.8 -0.78571429 -0.77142857 -0.75714286 -0.74285714 -0.72857143 -0.71428571 -0.7 -0.68571429 -0.67142857 -0.65714286 -0.64285714 -0.62857143 -0.61428571 -0.6 -0.58571429 -0.57142857 -0.55714286 -0.54285714 -0.52857143 -0.51428571 -0.5 -0.48571429 -0.47142857 -0.45714286 -0.44285714 -0.42857143 -0.41428571 -0.4 -0.38571429 -0.37142857 -0.35714286 -0.34285714 -0.32857143 -0.31428571 -0.3 -0.28571429 -0.27142857 -0.25714286 -0.24285714 -0.22857143 -0.21428571 -0.2 -0.18571429 -0.17142857 -0.15714286 -0.14285714 -0.12857143 -0.11428571 -0.1 -0.08571429 -0.07142857 -0.05714286 -0.04285714 -0.02857143 -0.01428571 0 0 0 0 0 0
  line L11 (1.7068, -18.7162) -> (1.6608, -18.2077)
  arc A23 (2.3091, -17.3966) -> (1.6608, -18.2077) centre (2.4078, -18.1401) ccw
  arc A24 (2.3091, -17.3966) -> (3.1798, -17.2587) centre (0, 0) ccw
  arc A25 (4.0469, -17.8298) -> (3.1798, -17.2587) centre (3.3157, -17.9963) ccw
  line L12 (4.0469, -17.8298) -> (4.1603, -18.3276)
  spline S12 degree 5 poles (4.1603, -18.3276) (4.1624, -18.3368) (4.1668, -18.3551) (4.1742, -18.3824) (4.1854, -18.4183) (4.2012, -18.4627) (4.2183, -18.5068) (4.2364, -18.5506) (4.2548, -18.5943) (4.2736, -18.6379) (4.2927, -18.6814) (4.3123, -18.7248) (4.3324, -18.7681) (4.3531, -18.8111) (4.3745, -18.8539) (4.3965, -18.8966) (4.419, -18.939) (4.442, -18.9813) (4.4653, -19.0235) (4.489, -19.0656) (4.5131, -19.1076) (4.5375, -19.1494) (4.5623, -19.1911) (4.5875, -19.2326) (4.6131, -19.274) (4.6391, -19.3153) (4.6654, -19.3564) (4.6921, -19.3974) (4.7192, -19.4383) (4.7465, -19.479) (4.7742, -19.5196) (4.8022, -19.5601) (4.8305, -19.6005) (4.8592, -19.6407) (4.8881, -19.6808) (4.9174, -19.7208) (4.9469, -19.7607) (4.9768, -19.8004) (5.0069, -19.84) (5.0374, -19.8795) (5.0681, -19.9188) (5.0991, -19.9581) (5.1304, -19.9972) (5.162, -20.0361) (5.1938, -20.075) (5.2259, -20.1137) (5.2583, -20.1523) (5.291, -20.1908) (5.3239, -20.2292) (5.3571, -20.2674) (5.3905, -20.3055) (5.4242, -20.3435) (5.4581, -20.3813) (5.4923, -20.4191) (5.5267, -20.4567) (5.5614, -20.4942) (5.5964, -20.5315) (5.6315, -20.5688) (5.6669, -20.6059) (5.7026, -20.6429) (5.7385, -20.6797) (5.7746, -20.7164) (5.811, -20.753) (5.8476, -20.7895) (5.8844, -20.8259) (5.9214, -20.8621) (5.9587, -20.8982) (5.9962, -20.9342) (6.0339, -20.97) (6.0718, -21.0057) (6.11, -21.0413) (6.1407, -21.0697) (6.1638, -21.0909) (6.1793, -21.105) (6.187, -21.1121) knots 0 0 0 0 0 0 0.01428571 0.02857143 0.04285714 0.05714286 0.07142857 0.08571429 0.1 0.11428571 0.12857143 0.14285714 0.15714286 0.17142857 0.18571429 0.2 0.21428571 0.22857143 0.24285714 0.25714286 0.27142857 0.28571429 0.3 0.31428571 0.32857143 0.34285714 0.35714286 0.37142857 0.38571429 0.4 0.41428571 0.42857143 0.44285714 0.45714286 0.47142857 0.48571429 0.5 0.51428571 0.52857143 0.54285714 0.55714286 0.57142857 0.58571429 0.6 0.61428571 0.62857143 0.64285714 0.65714286 0.67142857 0.68571429 0.7 0.71428571 0.72857143 0.74285714 0.75714286 0.77142857 0.78571429 0.8 0.81428571 0.82857143 0.84285714 0.85714286 0.87142857 0.88571429 0.9 0.91428571 0.92857143 0.94285714 0.95714286 0.97142857 0.98571429 1 1 1 1 1 1
  arc A26 (6.187, -21.1121) -> (7.404, -20.7167) centre (0, 0) ccw
  spline S13 degree 5 poles (7.404, -20.7167) (7.4061, -20.7064) (7.4103, -20.6859) (7.4165, -20.6552) (7.4247, -20.6142) (7.4346, -20.5629) (7.4443, -20.5117) (7.4538, -20.4606) (7.463, -20.4094) (7.4719, -20.3583) (7.4806, -20.3072) (7.489, -20.2562) (7.4972, -20.2052) (7.5051, -20.1542) (7.5127, -20.1032) (7.5201, -20.0523) (7.5272, -20.0014) (7.534, -19.9506) (7.5406, -19.8998) (7.5469, -19.8491) (7.5529, -19.7983) (7.5587, -19.7477) (7.5641, -19.6971) (7.5693, -19.6465) (7.5743, -19.5959) (7.5789, -19.5455) (7.5833, -19.495) (7.5874, -19.4447) (7.5912, -19.3943) (7.5947, -19.3441) (7.5979, -19.2939) (7.6008, -19.2437) (7.6034, -19.1936) (7.6058, -19.1436) (7.6078, -19.0936) (7.6095, -19.0437) (7.611, -18.9939) (7.6121, -18.9441) (7.6129, -18.8944) (7.6134, -18.8448) (7.6135, -18.7953) (7.6134, -18.7458) (7.6129, -18.6964) (7.6121, -18.6471) (7.6109, -18.5979) (7.6095, -18.5488) (7.6076, -18.4998) (7.6055, -18.4508) (7.603, -18.4019) (7.6001, -18.3532) (7.5969, -18.3045) (7.5933, -18.256) (7.5893, -18.2076) (7.5848, -18.1592) (7.58, -18.1111) (7.5748, -18.063) (7.5692, -18.015) (7.5633, -17.9672) (7.557, -17.9194) (7.5503, -17.8718) (7.543, -17.8244) (7.5351, -17.7772) (7.5266, -17.7302) (7.5175, -17.6834) (7.5078, -17.6368) (7.4976, -17.5904) (7.4872, -17.544) (7.4765, -17.4978) (7.4653, -17.4518) (7.4533, -17.4061) (7.44, -17.3608) (7.4279, -17.3252) (7.4178, -17.2988) (7.4106, -17.2814) (7.4069, -17.2727) knots -1 -1 -1 -1 -1 -1 -0.98571429 -0.97142857 -0.95714286 -0.94285714 -0.92857143 -0.91428571 -0.9 -0.88571429 -0.87142857 -0.85714286 -0.84285714 -0.82857143 -0.81428571 -0.8 -0.78571429 -0.77142857 -0.75714286 -0.74285714 -0.72857143 -0.71428571 -0.7 -0.68571429 -0.67142857 -0.65714286 -0.64285714 -0.62857143 -0.61428571 -0.6 -0.58571429 -0.57142857 -0.55714286 -0.54285714 -0.52857143 -0.51428571 -0.5 -0.48571429 -0.47142857 -0.45714286 -0.44285714 -0.42857143 -0.41428571 -0.4 -0.38571429 -0.37142857 -0.35714286 -0.34285714 -0.32857143 -0.31428571 -0.3 -0.28571429 -0.27142857 -0.25714286 -0.24285714 -0.22857143 -0.21428571 -0.2 -0.18571429 -0.17142857 -0.15714286 -0.14285714 -0.12857143 -0.11428571 -0.1 -0.08571429 -0.07142857 -0.05714286 -0.04285714 -0.02857143 -0.01428571 0 0 0 0 0 0
  line L13 (7.4069, -17.2727) -> (7.206, -16.8033)
  arc A27 (7.5719, -15.8316) -> (7.206, -16.8033) centre (7.8955, -16.5082) ccw
  arc A28 (7.5719, -15.8316) -> (8.3574, -15.4314) centre (0, 0) ccw
  arc A29 (9.3586, -15.7065) -> (8.3574, -15.4314) centre (8.7145, -16.0909) ccw
  line L14 (9.3586, -15.7065) -> (9.6202, -16.145)
  spline S14 degree 5 poles (9.6202, -16.145) (9.6251, -16.1531) (9.6349, -16.1691) (9.6504, -16.1928) (9.6721, -16.2235) (9.7009, -16.2609) (9.7308, -16.2974) (9.7615, -16.3336) (9.7925, -16.3694) (9.8239, -16.4051) (9.8555, -16.4406) (9.8875, -16.4758) (9.92, -16.5107) (9.953, -16.5452) (9.9866, -16.5793) (10.0207, -16.6131) (10.0552, -16.6465) (10.0902, -16.6797) (10.1254, -16.7126) (10.1609, -16.7453) (10.1967, -16.7778) (10.2329, -16.81) (10.2694, -16.842) (10.3062, -16.8737) (10.3433, -16.9052) (10.3808, -16.9364) (10.4186, -16.9673) (10.4566, -16.9981) (10.495, -17.0286) (10.5336, -17.0589) (10.5724, -17.089) (10.6116, -17.1188) (10.651, -17.1485) (10.6906, -17.1779) (10.7306, -17.2071) (10.7708, -17.2361) (10.8112, -17.2648) (10.8519, -17.2934) (10.8928, -17.3217) (10.9339, -17.3499) (10.9753, -17.3778) (11.0169, -17.4055) (11.0588, -17.433) (11.1008, -17.4604) (11.1431, -17.4875) (11.1857, -17.5144) (11.2284, -17.5411) (11.2713, -17.5676) (11.3145, -17.5939) (11.3578, -17.62) (11.4014, -17.6459) (11.4452, -17.6716) (11.4892, -17.6972) (11.5333, -17.7225) (11.5777, -17.7476) (11.6223, -17.7725) (11.667, -17.7973) (11.712, -17.8218) (11.7572, -17.8462) (11.8025, -17.8703) (11.848, -17.8943) (11.8937, -17.9181) (11.9396, -17.9416) (11.9857, -17.965) (12.0319, -17.9882) (12.0783, -18.0112) (12.1249, -18.034) (12.1717, -18.0567) (12.2187, -18.0791) (12.2658, -18.1013) (12.3131, -18.1234) (12.351, -18.1409) (12.3796, -18.1539) (12.3987, -18.1626) (12.4082, -18.1669) knots 0 0 0 0 0 0 0.01428571 0.02857143 0.04285714 0.05714286 0.07142857 0.08571429 0.1 0.11428571 0.12857143 0.14285714 0.15714286 0.17142857 0.18571429 0.2 0.21428571 0.22857143 0.24285714 0.25714286 0.27142857 0.28571429 0.3 0.31428571 0.32857143 0.34285714 0.35714286 0.37142857 0.38571429 0.4 0.41428571 0.42857143 0.44285714 0.45714286 0.47142857 0.48571429 0.5 0.51428571 0.52857143 0.54285714 0.55714286 0.57142857 0.58571429 0.6 0.61428571 0.62857143 0.64285714 0.65714286 0.67142857 0.68571429 0.7 0.71428571 0.72857143 0.74285714 0.75714286 0.77142857 0.78571429 0.8 0.81428571 0.82857143 0.84285714 0.85714286 0.87142857 0.88571429 0.9 0.91428571 0.92857143 0.94285714 0.95714286 0.97142857 0.98571429 1 1 1 1 1 1
  arc A30 (12.4082, -18.1669) -> (13.4434, -17.4148) centre (0, 0) ccw
  spline S15 degree 5 poles (13.4434, -17.4148) (13.4422, -17.4044) (13.4399, -17.3836) (13.4363, -17.3524) (13.4314, -17.3109) (13.4251, -17.2591) (13.4185, -17.2074) (13.4116, -17.1558) (13.4046, -17.1043) (13.3973, -17.053) (13.3897, -17.0017) (13.382, -16.9505) (13.374, -16.8995) (13.3657, -16.8486) (13.3572, -16.7978) (13.3485, -16.7471) (13.3395, -16.6965) (13.3303, -16.646) (13.3209, -16.5957) (13.3112, -16.5455) (13.3013, -16.4954) (13.2911, -16.4454) (13.2807, -16.3956) (13.27, -16.3459) (13.259, -16.2963) (13.2479, -16.2468) (13.2364, -16.1975) (13.2247, -16.1484) (13.2128, -16.0993) (13.2006, -16.0504) (13.1882, -16.0017) (13.1754, -15.9531) (13.1625, -15.9046) (13.1492, -15.8563) (13.1357, -15.8082) (13.1219, -15.7602) (13.1079, -15.7124) (13.0936, -15.6647) (13.079, -15.6172) (13.0641, -15.5698) (13.049, -15.5227) (13.0335, -15.4757) (13.0178, -15.4288) (13.0018, -15.3822) (12.9855, -15.3358) (12.9689, -15.2895) (12.952, -15.2434) (12.9349, -15.1975) (12.9174, -15.1518) (12.8996, -15.1063) (12.8815, -15.0611) (12.8631, -15.016) (12.8443, -14.9712) (12.8251, -14.9266) (12.8056, -14.8823) (12.7858, -14.8382) (12.7657, -14.7943) (12.7453, -14.7506) (12.7245, -14.7072) (12.7034, -14.664) (12.6819, -14.6211) (12.6598, -14.5786) (12.6372, -14.5366) (12.614, -14.4949) (12.5904, -14.4536) (12.5664, -14.4125) (12.5422, -14.3717) (12.5177, -14.331) (12.4928, -14.2907) (12.4673, -14.2509) (12.4406, -14.212) (12.4181, -14.1819) (12.4004, -14.1599) (12.3882, -14.1456) (12.382, -14.1385) knots -1 -1 -1 -1 -1 -1 -0.98571429 -0.97142857 -0.95714286 -0.94285714 -0.92857143 -0.91428571 -0.9 -0.88571429 -0.87142857 -0.85714286 -0.84285714 -0.82857143 -0.81428571 -0.8 -0.78571429 -0.77142857 -0.75714286 -0.74285714 -0.72857143 -0.71428571 -0.7 -0.68571429 -0.67142857 -0.65714286 -0.64285714 -0.62857143 -0.61428571 -0.6 -0.58571429 -0.57142857 -0.55714286 -0.54285714 -0.52857143 -0.51428571 -0.5 -0.48571429 -0.47142857 -0.45714286 -0.44285714 -0.42857143 -0.41428571 -0.4 -0.38571429 -0.37142857 -0.35714286 -0.34285714 -0.32857143 -0.31428571 -0.3 -0.28571429 -0.27142857 -0.25714286 -0.24285714 -0.22857143 -0.21428571 -0.2 -0.18571429 -0.17142857 -0.15714286 -0.14285714 -0.12857143 -0.11428571 -0.1 -0.08571429 -0.07142857 -0.05714286 -0.04285714 -0.02857143 -0.01428571 0 0 0 0 0 0
  line L15 (12.382, -14.1385) -> (12.0458, -13.7541)
  arc A31 (12.0936, -12.7169) -> (12.0458, -13.7541) centre (12.6104, -13.2604) ccw
  arc A32 (12.0936, -12.7169) -> (12.7169, -12.0936) centre (0, 0) ccw
  arc A33 (13.7541, -12.0458) -> (12.7169, -12.0936) centre (13.2604, -12.6104) ccw
  line L16 (13.7541, -12.0458) -> (14.1385, -12.382)
  spline S16 degree 5 poles (14.1385, -12.382) (14.1456, -12.3882) (14.1599, -12.4004) (14.1819, -12.4181) (14.212, -12.4406) (14.2509, -12.4673) (14.2907, -12.4928) (14.331, -12.5177) (14.3717, -12.5422) (14.4125, -12.5664) (14.4536, -12.5904) (14.4949, -12.614) (14.5366, -12.6372) (14.5786, -12.6598) (14.6211, -12.6819) (14.664, -12.7034) (14.7072, -12.7245) (14.7506, -12.7453) (14.7943, -12.7657) (14.8382, -12.7858) (14.8823, -12.8056) (14.9266, -12.8251) (14.9712, -12.8443) (15.016, -12.8631) (15.0611, -12.8815) (15.1063, -12.8996) (15.1518, -12.9174) (15.1975, -12.9349) (15.2434, -12.952) (15.2895, -12.9689) (15.3358, -12.9855) (15.3822, -13.0018) (15.4288, -13.0178) (15.4757, -13.0335) (15.5227, -13.049) (15.5698, -13.0641) (15.6172, -13.079) (15.6647, -13.0936) (15.7124, -13.1079) (15.7602, -13.1219) (15.8082, -13.1357) (15.8563, -13.1492) (15.9046, -13.1625) (15.9531, -13.1754) (16.0017, -13.1882) (16.0504, -13.2006) (16.0993, -13.2128) (16.1484, -13.2247) (16.1975, -13.2364) (16.2468, -13.2479) (16.2963, -13.259) (16.3459, -13.27) (16.3956, -13.2807) (16.4454, -13.2911) (16.4954, -13.3013) (16.5455, -13.3112) (16.5957, -13.3209) (16.646, -13.3303) (16.6965, -13.3395) (16.7471, -13.3485) (16.7978, -13.3572) (16.8486, -13.3657) (16.8995, -13.374) (16.9505, -13.382) (17.0017, -13.3897) (17.053, -13.3973) (17.1043, -13.4046) (17.1558, -13.4116) (17.2074, -13.4185) (17.2591, -13.4251) (17.3109, -13.4314) (17.3524, -13.4363) (17.3836, -13.4399) (17.4044, -13.4422) (17.4148, -13.4434) knots 0 0 0 0 0 0 0.01428571 0.02857143 0.04285714 0.05714286 0.07142857 0.08571429 0.1 0.11428571 0.12857143 0.14285714 0.15714286 0.17142857 0.18571429 0.2 0.21428571 0.22857143 0.24285714 0.25714286 0.27142857 0.28571429 0.3 0.31428571 0.32857143 0.34285714 0.35714286 0.37142857 0.38571429 0.4 0.41428571 0.42857143 0.44285714 0.45714286 0.47142857 0.48571429 0.5 0.51428571 0.52857143 0.54285714 0.55714286 0.57142857 0.58571429 0.6 0.61428571 0.62857143 0.64285714 0.65714286 0.67142857 0.68571429 0.7 0.71428571 0.72857143 0.74285714 0.75714286 0.77142857 0.78571429 0.8 0.81428571 0.82857143 0.84285714 0.85714286 0.87142857 0.88571429 0.9 0.91428571 0.92857143 0.94285714 0.95714286 0.97142857 0.98571429 1 1 1 1 1 1
  arc A34 (17.4148, -13.4434) -> (18.1669, -12.4082) centre (0, 0) ccw